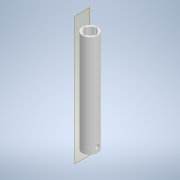
# Autodesk Inventor part: Soporte de Marcador
Saved by Autodesk Inventor 2022 (Build 260153000, 153)
## iProperties
Created: 2022-08-23
Part Number: Soporte de Marcador
Material: Generic
Document SubType Name: Modeling
Designer: David
Density: 1 g/cm^3
Appearance: Default
Author: David
Autodesk Inventor part; units mm, degrees
ref_plane "XZ Plane" through (0, 0, 0) normal (0, 1, 0) x (-1, 0, 0)
ref_plane "XY Plane" through (0, 0, 0) normal (0, 0, 1) x (1, 0, 0)
sketch "Sketch3" plane through (0, 0, 0) normal (1, 0, 0) x (0, 1, 0)
  line L0 (0, -2.6) -> (0, 15.6) projected
  line L1 (-33.9, 0) -> (203.4, 0) projected
  line L2 (0, 13) -> (169.5, 13)
  line L3 (169.5, 13) -> (169.5, 10)
  line L4 (169.5, 10) -> (25, 10)
  line L5 (25, 10) -> (25, 0)
  line L6 (0, 13) -> (0, 0)
  line L7 (25, 0) -> (0, 0)
  point P0 (0, 13)
  dimension "d10" = 169.5
  dimension "d13" = 10
  dimension "d14" = 13
  dimension "d15" = 25
  dimension "d17" = 3
  constraints: 12 end point, 2 collinear, 2 perpendicular, 1 horizontal, 1 point on line, 1 vertical
  measures "d10" distance of L2.start L2.end
  measures "d13" distance between parallel lines of L1 L4
  measures "d14" distance between parallel lines of L1 L2
  measures "d15" distance between parallel lines of L0 L5
  measures "d17" distance of L2.end L3.end
revolve "Revolution1" add sketch "Sketch3" angle 360 about axis through (0, -10, 0) along (0, 1, 0)
ref_plane "Work Plane1" through (-13, 84.75, 0) normal (1, 0, 0) x (0, 1, 0)
sketch "Sketch4" plane through (-13, 84.75, 0) normal (1, 0, 0) x (0, 1, 0)
  line L0 (-84.75, -13) -> (-84.75, 13) projected
  line L1 (-118.65, 0) -> (118.65, 0) projected
  point P0 (-84.75, 0)
  point P1 (-74.75, 0)
  dimension "d18" = 10
  constraints: 1 point on line
  measures "d18" distance from line of point (-74.75, 0) L0
hole "Hole1" at (-13, 10, 0) direction (1, 0, 0) diameter 6 end through all
sketch "Sketch5" plane through (0, 169.5, 0) normal (0, 1, 0) x (1, 0, 0)
  circle A0 centre (0, 0) radius 10 projected
  circle A1 centre (0, -10) radius 2.25
  line L0 (0, 18.2) -> (0, -18.2) projected
  point P0 (2.2357, -9.7469)
  point P1 (-2.2357, -9.7469)
  dimension "d26" = 4.5
  constraints: 1 centre point, 1 point on line, 2 other
  measures "d26" diameter of A1
extrude "Extrusion3" cut sketch "Sketch5" against normal up to surface (144.5 mm away) contours A1 L0 A0 | A0 L0 A1 picked at (0.5757, -10.6663) picked at (-0.5973, -10.6555)
pattern_circular "Circular Pattern1" count 4 over 360 about axis through (0, 97.25, 0) along (0, 1, 0) of "Extrusion3"
body "Solid2"
